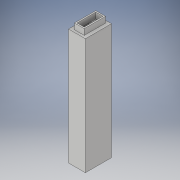
# Autodesk Inventor part: Bacon2
Saved by Autodesk Inventor 2018.2 (Build 222227000, 227)
## iProperties
Created: 2018-03-23
Part Number: Bacon2
Material: Generic
Document SubType Name: Modeling
Designer: MIABo
Density: 1 g/cm^3
Appearance: Default
Author: MIABo
Autodesk Inventor part; units mm, degrees
ref_plane "YZ Plane" through (0, 0, 0) normal (1, 0, 0) x (0, 1, 0)
ref_plane "XZ Plane" through (0, 0, 0) normal (0, 1, 0) x (-1, 0, 0)
ref_plane "XY Plane" through (0, 0, 0) normal (0, 0, 1) x (1, 0, 0)
sketch "Sketch1" plane through (0, 0, 0) normal (0, 1, 0) x (-1, 0, 0)
  line L0 (5.3975, 11.7221) -> (-5.3975, 11.7221)
  line L1 (-5.3975, 11.7221) -> (-5.3975, -11.7221)
  line L2 (-5.3975, -11.7221) -> (5.3975, -11.7221)
  line L3 (5.3975, -11.7221) -> (5.3975, 11.7221)
  line L4 (5.3975, 11.7221) -> (-5.3975, -11.7221) construction
  line L5 (-5.3975, 11.7221) -> (5.3975, -11.7221) construction
  line L6 (9.2075, 14.2621) -> (-9.2075, 14.2621)
  line L7 (-9.2075, 14.2621) -> (-9.2075, -14.2621)
  line L8 (-9.2075, -14.2621) -> (9.2075, -14.2621)
  line L9 (9.2075, -14.2621) -> (9.2075, 14.2621)
  line L10 (9.2075, 14.2621) -> (-9.2075, -14.2621) construction
  line L11 (-9.2075, 14.2621) -> (9.2075, -14.2621) construction
  point P0 (0, 0)
  dimension "d0" = 10.795
  dimension "d1" = 23.4442
  dimension "d2" = 18.415
  dimension "d3" = 28.5242
  constraints: 24 end point, 4 midpoint, 4 parallel, 2 horizontal, 2 perpendicular
  measures "d0" distance of L2.end L1.end
  measures "d1" distance of L1.end L0.end
  measures "d2" distance of L8.end L7.end
  measures "d3" distance of L7.end L6.end
extrude "Extrusion1" add sketch "Sketch1" along normal blind 127
sketch "Sketch2" plane through (0, 127, 0) normal (0, 1, 0) x (1, 0, 0)
  point P0 (0, 0)
sketch "Sketch3" plane through (0, 0, 0) normal (0, -1, 0) x (1, 0, 0)
  line L0 (5.3975, 11.7221) -> (5.3975, -11.7221) projected
  line L1 (-5.3975, 11.7221) -> (-5.3975, -11.7221) projected
  line L2 (5.3975, -11.7221) -> (-5.3975, -11.7221)
  line L3 (-5.3975, -11.7221) -> (-5.3975, -4.1021)
  line L4 (-5.3975, -4.1021) -> (5.3975, -4.1021)
  line L5 (5.3975, -4.1021) -> (5.3975, -11.7221)
  point P0 (0, 0)
  dimension "d6" = 7.62
  constraints: 8 end point, 2 parallel, 1 horizontal, 1 perpendicular, 1 point on line
  measures "d6" distance of L2.end L3.end
extrude "Extrusion2" add sketch "Sketch3" against normal blind 127
sketch "Sketch4" plane through (0, 127, 0) normal (0, 1, 0) x (1, 0, 0)
  line L0 (-5.3975, 11.7221) -> (5.3975, 11.7221)
  line L1 (5.3975, 11.7221) -> (5.3975, -11.7221)
  line L2 (5.3975, -11.7221) -> (-5.3975, -11.7221)
  line L3 (-5.3975, -11.7221) -> (-5.3975, 11.7221)
  line L4 (-5.3975, 11.7221) -> (5.3975, -11.7221) construction
  line L5 (5.3975, 11.7221) -> (-5.3975, -11.7221) construction
  line L6 (-3.8735, 10.1981) -> (3.8735, 10.1981)
  line L7 (3.8735, 10.1981) -> (3.8735, -10.1981)
  line L8 (3.8735, -10.1981) -> (-3.8735, -10.1981)
  line L9 (-3.8735, -10.1981) -> (-3.8735, 10.1981)
  line L10 (-3.8735, 10.1981) -> (3.8735, -10.1981) construction
  line L11 (3.8735, 10.1981) -> (-3.8735, -10.1981) construction
  point P0 (0, 0)
  dimension "d9" = 10.795
  dimension "d10" = 23.4442
  dimension "d11" = 7.747
  dimension "d12" = 20.3962
  constraints: 24 end point, 4 midpoint, 4 parallel, 2 horizontal, 2 perpendicular
  measures "d9" distance of L1.end L2.end
  measures "d10" distance of L0.end L1.end
  measures "d11" distance of L7.end L8.end
  measures "d12" distance of L6.end L7.end
extrude "Extrusion3" add sketch "Sketch4" along normal blind 6.35
body "Solid1"
